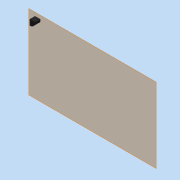
# Autodesk Inventor part: Part1
Saved by Autodesk Inventor 2017 (Build 210142000, 142)
## iProperties
Created: 2018-10-05
Part Number: Part1
Material: ABS Plastic
Document SubType Name: Modeling
Designer: mailb
Density: 1.06 g/cm^3
Appearance: Asphalt 2
Author: mailb
Autodesk Inventor part; units mm, degrees
ref_plane "YZ Plane" through (0, 0, 0) normal (1, 0, 0) x (0, 1, 0)
ref_plane "XZ Plane" through (0, 0, 0) normal (0, 1, 0) x (-1, 0, 0)
ref_plane "XY Plane" through (0, 0, 0) normal (0, 0, 1) x (1, 0, 0)
ref_plane "Work Plane1" through (0, 0, 0) normal (0, 0, 1) x (1, 0, 0)
sketch "Sketch1" plane through (0, 0, 0) normal (0, 0, 1) x (1, 0, 0)
  line L0 (-291.2125, -168.0875) -> (-291.2125, 168.0875) projected
  arc A0 (-291.2125, -168.0875) -> (-288.0375, -171.2625) centre (-288.0375, -168.0875) ccw projected
  line L1 (288.0375, -171.2625) -> (-288.0375, -171.2625) projected
  arc A1 (-288.0375, 171.2625) -> (-291.2125, 168.0875) centre (-288.0375, 168.0875) ccw projected
  line L2 (-288.0375, 171.2625) -> (288.0375, 171.2625) projected
  line L3 (-278.7, 142.24) -> (-278.7, 154.94) projected
  spline S0 degree 3 poles (-278.7, 154.94) (-278.7, 154.9595) (-278.6999, 154.979) (-278.6968, 155.1767) (-278.6816, 155.3543) (-278.6146, 155.7818) (-278.5502, 156.0273) (-278.2939, 156.7195) (-278.043, 157.129) (-277.3873, 157.8639) (-276.9741, 158.168) (-276.0102, 158.6259) (-275.4514, 158.75) (-274.89, 158.75) knots -0.643327 -0.643327 -0.643327 -0.643327 -0.63745 -0.63745 -0.583716 -0.583716 -0.506539 -0.506539 -0.357094 -0.357094 -0.190648 -0.190648 0 0 0 0 projected
  line L4 (-185.5704, 158.75) -> (-274.89, 158.75) projected
  line L5 (-278.7, 142.24) -> (-291.2125, 142.24)
  line L6 (-274.89, 158.75) -> (-262.19, 158.75)
  line L7 (-262.19, 158.75) -> (-262.19, 171.2625)
  point P0 (0, 0)
  dimension "d0" = 12.7
  constraints: 6 end point, 3 point on line, 2 perpendicular
  measures "d0" distance of L4.end L6.end
extrude "Extrusion1" add sketch "Sketch1" along normal blind 25.4
chamfer "Chamfer1" distance 3.175 angle 45 3 edges at (-277.5032, 157.7126, 25.4) (-268.54, 158.75, 25.4) (-278.7, 148.59, 25.4)
body "Solid1"
